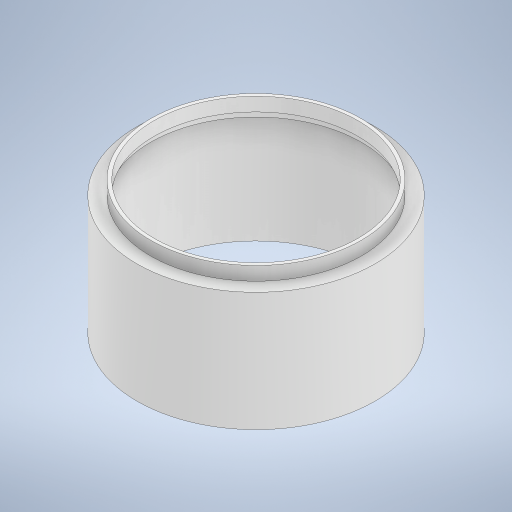
# Autodesk Inventor part: Parte media R2D2
Saved by Autodesk Inventor 2023 (Build 270158000, 158)
## iProperties
Created: 2022-10-09
Part Number: Parte media R2D2
Material: Generic
Document SubType Name: Modeling
Designer: User
Density: 1 g/cm^3
Appearance: Default
Author: User
Autodesk Inventor part; units mm, degrees
ref_plane "YZ Plane" through (0, 0, 0) normal (1, 0, 0) x (0, 1, 0)
ref_plane "XZ Plane" through (0, 0, 0) normal (0, 1, 0) x (-1, 0, 0)
ref_plane "XY Plane" through (0, 0, 0) normal (0, 0, 1) x (1, 0, 0)
sketch "Sketch1" plane through (0, 0, 0) normal (0, 1, 0) x (-1, 0, 0)
  circle A0 centre (0, 0) radius 175
  circle A1 centre (0, 0) radius 165
  dimension "d0" = 350
  dimension "d1" = 10
  constraints: 2 centre point, 2 coincident
  measures "d0" diameter of A0
  measures "d1" radial gap between concentric circles of A0 A1
extrude "Extrusion1" add sketch "Sketch1" along normal blind 175
sketch "Sketch2" plane through (0, 175, 0) normal (0, 1, 0) x (1, 0, 0)
  circle A0 centre (0, 0) radius 155
  circle A1 centre (0, 0) radius 150
  circle A2 centre (0, 0) radius 165 projected
  dimension "d4" = 10
  dimension "d5" = 5
  constraints: 2 centre point, 2 coincident
  measures "d4" radial gap between concentric circles of A2 A0
  measures "d5" radial gap between concentric circles of A0 A1
extrude "Extrusion2" add sketch "Sketch2" against normal blind 10 contours A2
extrude "Extrusion3" add sketch "Sketch2" along normal blind 20 contours A0
body "Solid1"
